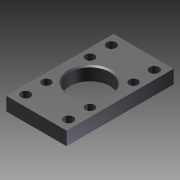
# Autodesk Inventor part: 174376 FNC-32---(F)
Saved by Autodesk Inventor 2011 SP1 (Build 150282100, 282)
## iProperties
Created: 2018-05-26
Part Number: 174376 FNC-32---(F)
Catalog Web Link: www.cadenas.de
Description: FNC-(F)-Flange mounting
Vendor: FESTO
Document SubType Name: Modeling
Designer: psAdmin
Manufacturer: FESTO
Mass: 24.9278 g
Surface Area: 105.474 cm^2
Volume: 24.9278 cm^3
Density: 1 g/cm^3
Category: PARTsolutions
Company: FESTO
Title: 174376 FNC-32
Author: Cadenas PARTsolutions
Comments: Flange mounting
PSOL_IDENT_0: {$CADENAS_DATA\23d-libs\festo\parts\f\fnc\fnc.prj},175 {VTYP=3D},{NB=174376 FNC-32---(F)},{LINA=1743
PSOL_IDENT_1: 76 FNC-32},{NN=FNC-(F)},{DATE=13.11.2017 12:35:20},{GEOMDATE=13.11.2017 12:34:23},{VERSION=},{LINEID=
PSOL_IDENT_2: 10},{LINESUBID=-1},{WBVAR=}  {NB=174376 FNC-32---(F)},{LINA=174376 FNC-32},{KT=DUMMY},{TNR=174376},{
PSOL_IDENT_3: TYP=FNC-32},{VERS=2},{D1=30.000},{D2=6.600},{D3=10.500},{E=45.000},{F=1.000},{FB=7.000},{MF=10.000},
PSOL_IDENT_4: {R=32.000},{T=5.000},{TF=64.000},{TG1=32.500},{UF=80.000},{ZZ=0},{DK=32},{D6912D=6.000},{D6912L=18.0
PSOL_IDENT_5: 00}
NN: FNC-(F)
NT: Flange mounting
NB: 174376 FNC-32---(F)
NBSYN: $TNR. $TYP.---(F)
LINA: 174376 FNC-32
TNR: 174376
TYP: FNC-32
D1: 30.000
D2: 6.600
D3: 10.500
E: 45.000
F: 1.000
FB: 7.000
MF: 10.000
R: 32.000
T: 5.000
TF: 64.000
TG1: 32.500
UF: 80.000
SUPPLIER: FESTO
ARTICLENO: 174376 FNC-32---(F)
BOMINFO: 174376 FNC-32
CREATOR: CADENAS GmbH
Autodesk Inventor part; units mm, degrees
sketch "Skizze_1" plane through (0, 0, 0) normal (0, 0, 1) x (1, 0, 0)
  line L0 (-22.5, 40) -> (-22.5, -40)
  line L1 (-22.5, -40) -> (22.5, -40)
  line L2 (22.5, -40) -> (22.5, 40)
  line L3 (22.5, 40) -> (-22.5, 40)
  circle A0 centre (16, 32) radius 3.5
  circle A1 centre (16, -32) radius 3.5
  circle A2 centre (-16, 32) radius 3.5
  circle A3 centre (-16, -32) radius 3.5
  constraints: 8 end point, 4 centre point
extrude "Extrusion1" add sketch "Skizze_1" along normal blind 10
sketch "Skizze_2_ALT_Drilling_1" plane through (0, 0, 0) normal (1, 0, 0) x (0, 1, 0)
  line L0 (0, 0) -> (0, 10)
  line L1 (0, 10) -> (16, 10)
  line L2 (16, 10) -> (15, 9)
  line L3 (15, 9) -> (15, 0)
  line L4 (15, 0) -> (0, 0)
  line L5 (0, 0) -> (0, 10)
  constraints: 12 end point
revolve "Revolution1" cut sketch "Skizze_2_ALT_Drilling_1" angle 360 about axis through (0, 0, 0) along (0, 0, -1)
sketch "Skizze_3_ALT_Drilling_2" plane through (16.25, 0, 0) normal (1, 0, 0) x (0, 0, -1)
  line L0 (0, 16.25) -> (-10, 16.25)
  line L1 (-10, 16.25) -> (-10, 19.55)
  line L2 (-10, 19.55) -> (-5, 19.55)
  line L3 (-5, 19.55) -> (-5, 21.5)
  line L4 (-5, 21.5) -> (0, 21.5)
  line L5 (0, 21.5) -> (0, 16.25)
  line L6 (0, 16.25) -> (-10, 16.25)
  constraints: 14 end point
revolve "Revolution2" cut sketch "Skizze_3_ALT_Drilling_2" angle 360 about axis through (16.25, 16.25, 0) along (0, 0, -1)
sketch "Muster_1_SKETCH_1" plane through (-16.25, 0, 0) normal (1, 0, 0) x (0, 0, -1)
  line L0 (0, 16.25) -> (-10, 16.25)
  line L1 (-10, 16.25) -> (-10, 19.55)
  line L2 (-10, 19.55) -> (-5, 19.55)
  line L3 (-5, 19.55) -> (-5, 21.5)
  line L4 (-5, 21.5) -> (0, 21.5)
  line L5 (0, 21.5) -> (0, 16.25)
  line L6 (0, 16.25) -> (-10, 16.25)
  constraints: 14 end point
sketch "Muster_1_SKETCH_2" plane through (16.25, 0, 0) normal (1, 0, 0) x (0, 0, -1)
  line L0 (0, -16.25) -> (-10, -16.25)
  line L1 (-10, -16.25) -> (-10, -12.95)
  line L2 (-10, -12.95) -> (-5, -12.95)
  line L3 (-5, -12.95) -> (-5, -11)
  line L4 (-5, -11) -> (0, -11)
  line L5 (0, -11) -> (0, -16.25)
  line L6 (0, -16.25) -> (-10, -16.25)
  constraints: 14 end point
sketch "Muster_1_SKETCH_3" plane through (-16.25, 0, 0) normal (1, 0, 0) x (0, 0, -1)
  line L0 (0, -16.25) -> (-10, -16.25)
  line L1 (-10, -16.25) -> (-10, -12.95)
  line L2 (-10, -12.95) -> (-5, -12.95)
  line L3 (-5, -12.95) -> (-5, -11)
  line L4 (-5, -11) -> (0, -11)
  line L5 (0, -11) -> (0, -16.25)
  line L6 (0, -16.25) -> (-10, -16.25)
  constraints: 14 end point
revolve "Revolution3" cut sketch "Muster_1_SKETCH_1" angle 360 about axis through (-16.25, 16.25, 0) along (0, 0, -1)
revolve "Revolution4" cut sketch "Muster_1_SKETCH_2" angle 360 about axis through (16.25, -16.25, 0) along (0, 0, -1)
revolve "Revolution5" cut sketch "Muster_1_SKETCH_3" angle 360 about axis through (-16.25, -16.25, 0) along (0, 0, -1)
ref_plane "FDT_MOUNT_XY" through (0, 0, 10) normal (0, 0, 1) x (0, 1, 0)
ref_plane "FDT_MOUNT_YZ" through (0, 0, 10) normal (0, 1, 0) x (-1, 0, 0)
ref_plane "FDT_MOUNT_ZX" through (0, 0, 10) normal (-1, 0, 0) x (0, 0, 1)
ref_plane "FNC_1_XY" through (0, 0, 5) normal (0, 0, 1) x (1, 0, 0)
ref_plane "FNC_1_YZ" through (0, 0, 5) normal (1, 0, 0) x (0, 1, 0)
ref_plane "FNC_1_ZX" through (0, 0, 5) normal (0, 1, 0) x (0, 0, 1)
ref_plane "FNC_2_3_XY" through (0, 0, 10) normal (0, 0, 1) x (1, 0, 0)
ref_plane "FNC_2_3_YZ" through (0, 0, 10) normal (1, 0, 0) x (0, 1, 0)
ref_plane "FNC_2_3_ZX" through (0, 0, 10) normal (0, 1, 0) x (0, 0, 1)
ref_plane "FNC_Schraube_1_XY" through (-16.25, 16.25, 5) normal (0, 0, 1) x (1, 0, 0)
ref_plane "FNC_Schraube_1_YZ" through (-16.25, 16.25, 5) normal (1, 0, 0) x (0, 1, 0)
ref_plane "FNC_Schraube_1_ZX" through (-16.25, 16.25, 5) normal (0, 1, 0) x (0, 0, 1)
ref_plane "FNC_Schraube_2_XY" through (16.25, 16.25, 5) normal (0, 0, 1) x (1, 0, 0)
ref_plane "FNC_Schraube_2_YZ" through (16.25, 16.25, 5) normal (1, 0, 0) x (0, 1, 0)
ref_plane "FNC_Schraube_2_ZX" through (16.25, 16.25, 5) normal (0, 1, 0) x (0, 0, 1)
ref_plane "FNC_Schraube_3_XY" through (-16.25, -16.25, 5) normal (0, 0, 1) x (1, 0, 0)
ref_plane "FNC_Schraube_3_YZ" through (-16.25, -16.25, 5) normal (1, 0, 0) x (0, 1, 0)
ref_plane "FNC_Schraube_3_ZX" through (-16.25, -16.25, 5) normal (0, 1, 0) x (0, 0, 1)
ref_plane "FNC_Schraube_4_XY" through (16.25, -16.25, 5) normal (0, 0, 1) x (1, 0, 0)
ref_plane "FNC_Schraube_4_YZ" through (16.25, -16.25, 5) normal (1, 0, 0) x (0, 1, 0)
ref_plane "FNC_Schraube_4_ZX" through (16.25, -16.25, 5) normal (0, 1, 0) x (0, 0, 1)
ref_plane "P17_XY" through (16, 32, 10) normal (0, 0, 1) x (1, 0, 0)
ref_plane "P17_YZ" through (16, 32, 10) normal (1, 0, 0) x (0, 1, 0)
ref_plane "P17_ZX" through (16, 32, 10) normal (0, 1, 0) x (0, 0, 1)
ref_plane "P18_XY" through (16, -32, 10) normal (0, 0, 1) x (1, 0, 0)
ref_plane "P18_YZ" through (16, -32, 10) normal (1, 0, 0) x (0, 1, 0)
ref_plane "P18_ZX" through (16, -32, 10) normal (0, 1, 0) x (0, 0, 1)
ref_plane "P19_XY" through (-16, -32, 10) normal (0, 0, 1) x (1, 0, 0)
ref_plane "P19_YZ" through (-16, -32, 10) normal (1, 0, 0) x (0, 1, 0)
ref_plane "P19_ZX" through (-16, -32, 10) normal (0, 1, 0) x (0, 0, 1)
ref_plane "P20_XY" through (-16, 32, 10) normal (0, 0, 1) x (1, 0, 0)
ref_plane "P20_YZ" through (-16, 32, 10) normal (1, 0, 0) x (0, 1, 0)
ref_plane "P20_ZX" through (-16, 32, 10) normal (0, 1, 0) x (0, 0, 1)
body "Solid1"
